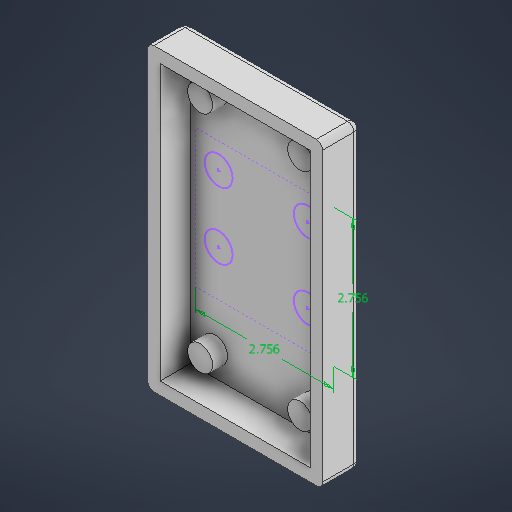
# Autodesk Inventor part: Bottom_Shell
Saved by Autodesk Inventor 2026.2 (Build 302298010, 298A)
## iProperties
Created: 2026-03-03
Part Number: Bottom_Shell
Material: Generic
Document SubType Name: Modeling
Designer: kjedr
Density: 1 g/cm^3
Appearance: Default
Author: kjedr
Autodesk Inventor part; units mm, degrees
ref_plane "YZ Plane" through (0, 0, 0) normal (1, 0, 0) x (0, 1, 0)
ref_plane "XZ Plane" through (0, 0, 0) normal (0, 1, 0) x (-1, 0, 0)
ref_plane "XY Plane" through (0, 0, 0) normal (0, 0, 1) x (1, 0, 0)
sketch "Sketch1" plane through (0, 0, 0) normal (0, 0, 1) x (1, 0, 0)
  line L0 (0, 0) -> (88.9, 0)
  line L1 (88.9, 0) -> (88.9, 152.4)
  line L2 (88.9, 152.4) -> (0, 152.4)
  line L3 (0, 152.4) -> (0, 0)
  dimension "d0" = 88.9
  dimension "d1" = 152.4
  constraints: 8 end point, 2 parallel, 1 horizontal, 1 perpendicular
  measures "d0" distance of L2.end L1.end
  measures "d1" distance of L1.end L0.end
extrude "Extrusion1" add sketch "Sketch1" along normal blind 19.05
sketch "Sketch2" plane through (0, 0, 19.05) normal (0, 0, 1) x (1, 0, 0)
  line L0 (6.35, 6.35) -> (82.55, 6.35)
  line L1 (82.55, 6.35) -> (82.55, 146.05)
  line L2 (82.55, 146.05) -> (6.35, 146.05)
  line L3 (6.35, 146.05) -> (6.35, 6.35)
  line L4 (0, 152.4) -> (0, 0) projected
  line L5 (0, 0) -> (88.9, 0) projected
  line L6 (88.9, 0) -> (88.9, 152.4) projected
  line L7 (88.9, 152.4) -> (0, 152.4) projected
  point P0 (88.9, 76.2)
  dimension "d4" = 6.35
  dimension "d5" = 6.35
  dimension "d6" = 6.35
  dimension "d7" = 6.35
  constraints: 8 end point, 2 parallel, 1 horizontal, 1 midpoint, 1 perpendicular
  measures "d4" distance between parallel lines of L4 L3
  measures "d5" distance between parallel lines of L5 L0
  measures "d6" distance from line of point (88.9, 76.2) L1
  measures "d7" distance between parallel lines of L7 L2
extrude "Extrusion2" cut sketch "Sketch2" against normal blind 15.24 contours L3 L2 L1 L0
fillet "Fillet1" radius 3.175 8 edges at (44.45, 152.4, 0) (88.9, 76.2, 0) (88.9, 0, 9.525) (0, 76.2, 0) (44.45, 0, 0) (88.9, 152.4, 9.525) (0, 152.4, 9.525) (0, 0, 9.525)
sketch "Sketch5" plane through (0, 0, 3.81) normal (0, 0, 1) x (1, 0, 0)
  circle A0 centre (19.05, 133.35) radius 6.35
  circle A1 centre (69.85, 133.35) radius 6.35
  circle A2 centre (19.05, 19.05) radius 6.35
  circle A3 centre (69.85, 19.05) radius 6.35
  line L0 (6.35, 6.35) -> (6.35, 146.05) projected
  line L1 (6.35, 146.05) -> (82.55, 146.05) projected
  line L2 (82.55, 146.05) -> (82.55, 6.35) projected
  line L3 (82.55, 6.35) -> (6.35, 6.35) projected
  point P0 (0, 0)
  dimension "d11" = 12.7
  dimension "d12" = 12.7
  dimension "d13" = 12.7
  dimension "d14" = 12.7
  dimension "d15" = 12.7
  constraints: 4 centre point, 3 equal radius, 2 horizontal alignment, 2 vertical alignment
  measures "d11" diameter of A0
  measures "d12" distance from line of L0 A0.centre
  measures "d13" distance from line of L1 A0.centre
  measures "d14" distance from line of L2 A1.centre
  measures "d15" distance from line of L3 A3.centre
extrude "Extrusion3" add sketch "Sketch5" along normal blind 7.62 contours A0 | A1 | A2 | A3
sketch "Sketch6" plane through (0, 0, 3.81) normal (0, 0, 1) x (1, 0, 0)
  line L0 (9.0883, 111.6429) -> (79.0883, 111.6429) construction
  line L1 (79.0883, 111.6429) -> (79.0883, 41.6429) construction
  line L2 (79.0883, 41.6429) -> (9.0883, 41.6429) construction
  line L3 (9.0883, 41.6429) -> (9.0883, 111.6429) construction
  circle A0 centre (20.846, 98.7818) radius 7.1135
  circle A1 centre (66.1306, 98.7818) radius 7.1135
  circle A2 centre (20.846, 64.984) radius 7.1135
  circle A3 centre (66.1306, 60.566) radius 7.1135
  point P0 (0, 0)
  dimension "d18" = 70
  dimension "d19" = 70
  constraints: 8 end point, 4 centre point, 3 equal radius, 2 parallel, 1 horizontal, 1 perpendicular
  measures "d18" distance of L1.end L2.end
  measures "d19" distance of L0.end L1.end
body "Solid1"
